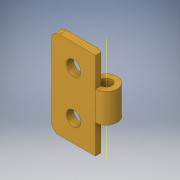
# Autodesk Inventor part: hinge right
Saved by Autodesk Inventor 2016 (Build 200138000, 138)
## iProperties
Created: 2017-11-05
Part Number: hinge right
Material: Brass, Soft Yellow
Document SubType Name: Modeling
Designer: mathaetaes
Density: 8.47 g/cm^3
Appearance: Brass - Satin
Author: mathaetaes
Autodesk Inventor part; units mm, degrees
ref_plane "YZ Plane" through (0, 0, 0) normal (1, 0, 0) x (0, 1, 0)
ref_plane "XZ Plane" through (0, 0, 0) normal (0, 1, 0) x (-1, 0, 0)
sketch "Sketch1" plane through (0, 0, 0) normal (0, 0, 1) x (1, 0, 0)
  line L0 (0, 12.0154) -> (19.05, 12.0154)
  line L1 (19.05, 12.0154) -> (19.05, -26.0846)
  line L2 (19.05, -26.0846) -> (0, -26.0846)
  line L3 (0, -26.0846) -> (0, 12.0154)
  circle A0 centre (9.525, 2.4904) radius 3.175
  circle A1 centre (9.525, -16.5596) radius 3.175
  point P0 (0, 0)
  dimension "d0" = 19.05
  dimension "d1" = 38.1
  dimension "d2" = 6.35
  dimension "d3" = 6.35
  dimension "d4" = 19.05
  dimension "d5" = 9.525
  dimension "d6" = 9.525
  constraints: 8 end point, 2 centre point, 2 parallel, 1 horizontal, 1 perpendicular
  measures "d0" distance of L1.end L2.end
  measures "d1" distance of L0.end L1.end
  measures "d2" diameter of A0
  measures "d3" diameter of A1
  measures "d4" distance of A1.centre A0.centre
  measures "d5" distance from line of L0 A0.centre
  measures "d6" distance from line of L3 A0.centre
extrude "Extrusion1" add sketch "Sketch1" along normal blind 3.175
fillet "Fillet1" radius 3.175 2 edges at (0, 12.0154, 1.5875) (0, -26.0846, 1.5875)
ref_plane "Work Plane1" through (3.175, -7.0346, 3.175) normal (0, 1, 0) x (1, 0, 0)
sketch "Sketch3" plane through (3.175, -7.0346, 3.175) normal (0, 1, 0) x (1, 0, 0)
  circle A0 centre (15.875, 4.7625) radius 4.7625
  line L0 (0, 3.175) -> (15.875, 3.175) projected
  line L1 (15.875, 0) -> (0, 0) projected
  point P0 (-3.175, 3.175)
  dimension "d21" = 9.525
  constraints: 1 centre point, 1 tangent
  measures "d21" diameter of A0
extrude "Extrusion4" add sketch "Sketch3" along normal mid plane 12.7
sketch "Sketch6" plane through (19.05, 12.0154, 3.175) normal (0, 1, 0) x (1, 0, 0)
  circle A0 centre (0, 4.7625) radius 2.3813
  arc A1 (0, 0) -> (-4.4901, 3.175) centre (0, 4.7625) ccw projected
  point P0 (-19.05, 3.175)
  point P1 (-4.4901, 0)
  point P2 (0, 3.175)
  dimension "d18" = 4.7625
  constraints: 1 centre point, 2 other
  measures "d18" diameter of A0
extrude "Extrusion5" cut sketch "Sketch6" against normal blind 38.1
sketch "Sketch8" plane through (0, 0, 0) normal (0, 1, 0) x (-1, 0, 0)
  arc A0 (-19.05, 0.7937) -> (-17.2751, 0) centre (-19.05, -1.5875) ccw projected
  line L0 (-14.5599, 0) -> (-17.2751, 0) projected
  arc A1 (-19.05, 3.175) -> (-14.5599, 0) centre (-19.05, -1.5875) ccw projected
  line L1 (-19.05, 0.7937) -> (-19.05, 3.175) projected
  line L2 (-3.175, 3.175) -> (0, 3.175) projected
  line L3 (0, 3.175) -> (0, 0) projected
  line L4 (0, 0) -> (-3.175, 0) projected
  line L5 (-3.175, 0) -> (-3.175, 3.175) projected
  line L6 (0, 0) -> (-14.2875, 0)
  line L7 (-14.2875, 0) -> (-14.2875, -6.4324)
  line L8 (-14.2875, -6.4324) -> (0, -6.4324)
  line L9 (0, -6.4324) -> (0, 0)
  dimension "d22" = 14.2875
  constraints: 8 end point, 2 parallel, 1 horizontal, 1 perpendicular, 1 tangent
  measures "d22" distance of L7.end L8.end
equation "\"d3\" = d2"
equation "\"d4\" = 0.5 * d1"
equation "\"d5\" = 0.25 * d1"
equation "\"d6\" = 0.5 * d0"
body "Solid1"
